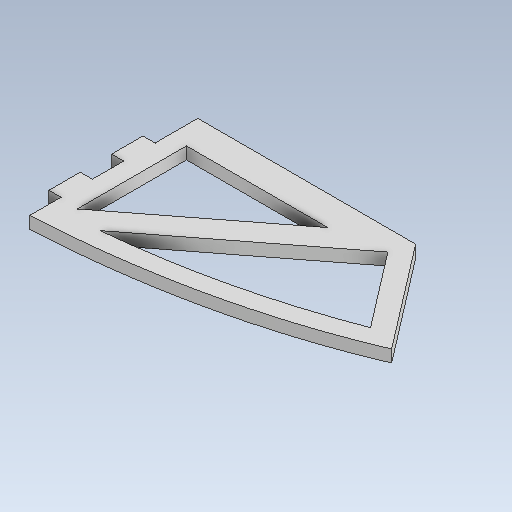
# Autodesk Inventor part: bulkhead_F2
Saved by Autodesk Inventor 2020.3 (Build 243373010, 373A)
## iProperties
Created: 2020-05-22
Part Number: bulkhead_F2
Material: Generic
Document SubType Name: Modeling
Designer: kardo
Density: 1 g/cm^3
Appearance: Default
Mass: 1.14831 g
Surface Area: 17.4945 cm^2
Volume: 1.14831 cm^3
Author: kardo
Autodesk Inventor part; units mm, degrees
ref_plane "YZ Plane" through (0, 0, 0) normal (1, 0, 0) x (0, 1, 0)
ref_plane "XZ Plane" through (0, 0, 0) normal (0, 1, 0) x (-1, 0, 0)
ref_plane "XY Plane" through (0, 0, 0) normal (0, 0, 1) x (1, 0, 0)
derived "base_sketch.ipt"
sketch "bulkhead_F2" plane through (0, 158.1, 33.6972) normal (0, 1, 0) x (-1, 0, 0)
  line L0 (19.176, 13.1208) -> (62.322, 13.1208)
  line L1 (62.322, 13.1208) -> (62.322, -20.1682)
  line L2 (0, -33.6972) -> (-11.5056, -33.6972)
  line L3 (-11.5056, -36.1839) -> (-34.5168, -36.1839)
  line L4 (-11.5056, -33.6972) -> (-11.5056, -36.1839)
  line L5 (-34.5168, -36.1839) -> (-57.528, -6.1572)
  line L6 (0, 5.8272) -> (0, -20.0113)
  line L7 (0, -20.0113) -> (-11.5056, -20.0113)
  line L8 (-11.5056, -20.0113) -> (-11.5056, -21.8764)
  line L9 (-11.5056, -21.8764) -> (-35.9142, -21.8764)
  line L10 (-35.9142, -21.8764) -> (-48.8988, -4.9332)
  line L11 (-57.528, -8.9984) -> (-57.528, -6.1572) construction
  line L12 (-33.1694, 4.9025) -> (-33.1694, 0.5647) construction
  line L13 (-16.7797, 9.4385) -> (-16.7797, 4.0937) construction
  line L14 (0, 12.2028) -> (0, 5.8272) construction
  spline S0 degree 4 poles (-57.528, -6.1572) (-46.0483, 0.508) (-30.6129, 6.8309) (-11.2214, 11.3442) (8.3201, 13.1208) (15.5662, 13.1208) (19.176, 13.1208) knots 0 0 0 0 0 0.630279 0.815816 1 1 1 1 1
  spline S1 degree 3 poles (-48.8988, -4.9332) (-33.5177, 1.6364) (-16.8054, 4.937) (0, 5.8272) knots 0 0 0 0 1 1 1 1
  line L15 (0, 2.0028) -> (-57.528, -6.1572) construction
  line L16 (0, 19.4965) -> (0, 13.1208) construction
  line L17 (0, 13.1208) -> (-57.528, 13.1208) construction
  line L18 (-57.528, 13.1208) -> (-57.528, 15.9621) construction
  line L19 (-57.528, 15.9621) -> (0, 19.4965) construction
  line L20 (-33.1694, 17.4586) -> (-33.1694, 13.1208) construction
  line L21 (-16.7797, 18.4656) -> (-16.7797, 13.1208) construction
  line L22 (-48.8988, -4.9332) -> (-48.8988, -1.5617) construction
  line L23 (-48.8988, 16.4923) -> (-48.8988, 13.1208) construction
  line L24 (-11.5056, -21.8764) -> (0, -21.8764) construction
  line L25 (0, -21.8764) -> (0, -20.0113) construction
  line L26 (-48.8988, -1.5617) -> (-33.1694, 4.9025) construction
  line L27 (-33.1694, 4.9025) -> (-16.7797, 9.4385) construction
  line L28 (-16.7797, 9.4385) -> (0, 12.2028) construction
  spline S2 degree 3 poles (-57.528, -8.9984) (-54.6767, -7.5178) (-51.7989, -6.1654) (-48.8988, -4.9332) knots 0 0 0 0 1 1 1 1
  point P0 (-38.352, 3.0228)
  point P1 (-19.176, 8.898)
ref_plane "bulkhead_F2_plane" through (0, 158.1, 33.6972) normal (0, 1, 0) x (-1, 0, 0)
sketch "Sketch2" plane through (0, 158.1, 33.6972) normal (0, 1, 0) x (-1, 0, 0)
  spline S0 degree 3 poles (-48.8988, -4.9332) (-33.5177, 1.6364) (-16.8054, 4.937) (0, 5.8272) knots 0 0 0 0 1 1 1 1 projected
  line L0 (-35.9142, -21.8764) -> (-48.8988, -4.9332) projected
  line L1 (-11.5056, -21.8764) -> (-35.9142, -21.8764) projected
  line L2 (-11.5056, -20.0113) -> (-11.5056, -21.8764) projected
  line L3 (0, -20.0113) -> (-11.5056, -20.0113) projected
  line L4 (-44.1274, -6.2273) -> (-34.7554, -18.4566)
  line L5 (-34.7554, -18.4566) -> (-7.971, 2.2044)
  line L6 (-35.9142, -21.8764) -> (0, 5.8272) construction
  line L7 (-26.3328, -17.0113) -> (-3, -17.0113)
  line L8 (-3, -17.0113) -> (-3, 0.9871)
  line L9 (-3, 0.9871) -> (-26.3328, -17.0113)
  line L10 (0, 0.6595) -> (2, 0.6595)
  line L11 (2, 0.6595) -> (2, -4.5082)
  line L12 (2, -4.5082) -> (0, -4.5082)
  line L13 (0, -9.6759) -> (2, -9.6759)
  line L14 (2, -9.6759) -> (2, -14.8436)
  line L15 (2, -14.8436) -> (0, -14.8436)
  spline S1 degree 2 poles (-44.1274, -6.2273) (-26.6164, 0.4206) (-7.971, 2.2044) knots 0 0 0 1 1 1
  line L16 (-44.1274, -6.2273) -> (-45.214, -3.4311) construction
  line L17 (-26.3328, -0.7954) -> (-27.0038, 2.1286) construction
  line L18 (-7.971, 2.2044) -> (-8.2751, 5.1889) construction
  line L19 (-44.1274, -6.2273) -> (-26.3328, -0.7954) construction
  line L20 (-26.3328, -0.7954) -> (-7.971, 2.2044) construction
  line L21 (0, 0.6595) -> (0, 5.8272)
  line L22 (0, -4.5082) -> (0, -9.6759)
  line L23 (0, -14.8436) -> (0, -20.0113)
  line L24 (-11.5056, -21.8764) -> (0, -21.8764)
  line L25 (0, -21.8764) -> (0, -20.0113)
  point P0 (0, -33.6972)
  point P1 (-57.528, -8.9984)
  dimension "d1" = 4
  dimension "d2" = 3
  dimension "d4" = 3
  dimension "d5" = 3
  dimension "d6" = 2
  dimension "d7" = 3
  constraints: 44 end point, 7 equal length, 6 collinear, 4 horizontal, 4 parallel, 2 vertical, 10 other
  measures "d1" distance between parallel lines of L9 L5
  measures "d2" distance between parallel lines of L3 L7
  measures "d4" distance between parallel lines of L0 L4
  measures "d5" distance of L4.start L16.end
  measures "d6" distance of L14.end L15.end
  measures "d7" distance between parallel lines of L22 L8
extrude "Extrusion1" add sketch "Sketch2" along normal blind 2
equation "\"d6\" = stringer_thickness"
equation "\"d8\" = bulkhead_thickness"
equation "\"stringer_thickness\" = 2"
equation "\"bulkhead_thickness\" = 2"
body "Solid1"
